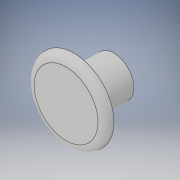
# Autodesk Inventor part: pin
Saved by Autodesk Inventor 2019 (Build 230136000, 136)
## iProperties
Created: 2020-02-07
Part Number: pin
Material: Generic
Document SubType Name: Modeling
Designer: Hugo Albarracin
Density: 1 g/cm^3
Appearance: Default
Author: Hugo Albarracin
Autodesk Inventor part; units mm, degrees
ref_plane "YZ Plane" through (0, 0, 0) normal (1, 0, 0) x (0, 1, 0)
ref_plane "XZ Plane" through (0, 0, 0) normal (0, 1, 0) x (-1, 0, 0)
ref_plane "XY Plane" through (0, 0, 0) normal (0, 0, 1) x (1, 0, 0)
sketch "Sketch2" plane through (0, 0, 0) normal (1, 0, 0) x (0, 1, 0)
  line L0 (0, 0) -> (5, 0)
  line L1 (5, 0) -> (5, -1)
  line L2 (5, -1) -> (2.5, -1)
  line L3 (2.5, -1) -> (2.5, -6)
  line L4 (2.5, -6) -> (0, -6)
  line L5 (0, -6) -> (0, 0)
  dimension "d0" = 5
  dimension "d1" = 1
  dimension "d2" = 2.5
  dimension "d3" = 5
  constraints: 12 end point, 5 perpendicular, 1 horizontal
  measures "d0" distance of L0.start L0.end
  measures "d1" distance of L0.end L1.end
  measures "d2" distance of L3.end L4.end
  measures "d3" distance of L2.end L3.end
revolve "Revolution1" add sketch "Sketch2" angle 360 about axis through (0, 0, -6) along (0, 0, 1)
fillet "Fillet1" radius 1 1 edges at (0, -5, 0)
body "Solid1"
